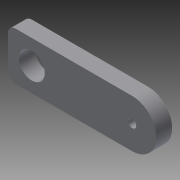
# Autodesk Inventor part: arm
Saved by Autodesk Inventor 2015 SP1 (Build 190203100, 203)
## iProperties
Created: 2016-02-02
Part Number: arm
Material: Generic
Document SubType Name: Modeling
Designer: tuttlem
Density: 1 g/cm^3
Appearance: Default
Author: tuttlem
Autodesk Inventor part; units mm, degrees
ref_plane "YZ Plane" through (0, 0, 0) normal (1, 0, 0) x (0, 1, 0)
ref_plane "XZ Plane" through (0, 0, 0) normal (0, 1, 0) x (-1, 0, 0)
ref_plane "XY Plane" through (0, 0, 0) normal (0, 0, 1) x (1, 0, 0)
sketch "Sketch1" plane through (0, 0, 0) normal (0, 0, 1) x (1, 0, 0)
  line L0 (-85.0546, 35.3436) -> (-85.0546, -40.8564)
  line L1 (-85.0546, -2.7564) -> (-46.9546, -2.7564)
  circle A0 centre (-46.9546, -2.7564) radius 20.6375
  line L2 (-46.9546, -2.7564) -> (113.0654, -2.7564)
  circle A1 centre (113.0654, -2.7564) radius 6.35
  line L3 (-85.0546, 35.3436) -> (113.0654, 35.3436)
  line L4 (-85.0546, -40.8564) -> (113.0654, -40.8564)
  arc A2 (113.0654, -40.8564) -> (113.0654, 35.3436) centre (113.0654, -2.7564) ccw
  point P0 (0, 0)
  point P1 (106.7321, -3.216)
  point P2 (113.0654, -3.216)
  dimension "d0" = 76.2
  dimension "d3" = 38.1
  dimension "d4" = 41.275
  dimension "d5" = 160.02
  dimension "d6" = 12.7
  constraints: 10 end point, 3 centre point, 3 coincident, 3 horizontal, 2 point on circle, 1 midpoint, 1 parallel, 1 vertical, 1 vertical alignment
  measures "d0" distance of L0.start L0.end
  measures "d3" distance of L1.start L1.end
  measures "d4" diameter of A0
  measures "d5" distance of L2.start L2.end
  measures "d6" diameter of A1
extrude "Extrusion1" add sketch "Sketch1" along normal blind 25.4
fillet "Fillet1" radius 12.7 2 edges at (-85.0546, 35.3436, 12.7) (-85.0546, -40.8564, 12.7)
body "Solid1"
